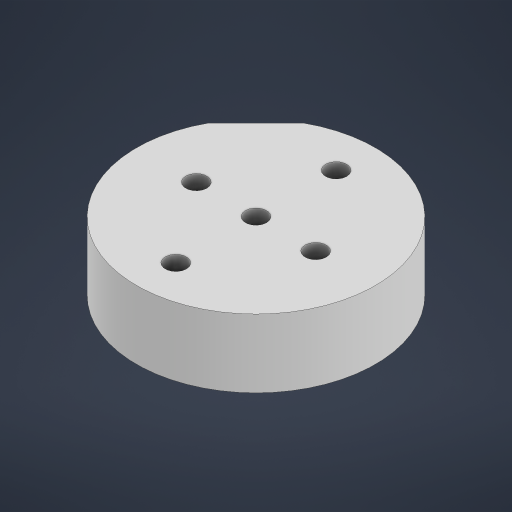
# Autodesk Inventor part: Pulley-35
Saved by Autodesk Inventor 2023 (Build 270158000, 158)
## iProperties
Created: 2023-09-04
Part Number: Pulley-35
Material: Generic
Document SubType Name: Modeling
Designer: Abhinav
Density: 1 g/cm^3
Appearance: Default
Author: Abhinav
Autodesk Inventor part; units mm, degrees
ref_plane "YZ Plane" through (0, 0, 0) normal (1, 0, 0) x (0, 1, 0)
ref_plane "XZ Plane" through (0, 0, 0) normal (0, 1, 0) x (-1, 0, 0)
ref_plane "XY Plane" through (0, 0, 0) normal (0, 0, 1) x (1, 0, 0)
sketch "Sketch1" plane through (0, 0, 0) normal (0, 1, 0) x (-1, 0, 0)
  line L0 (0, 0) -> (0, -11.75) construction
  circle A0 centre (0, -11.75) radius 1.55
  line L1 (0, 0) -> (8.75, 0) construction
  circle A1 centre (8.75, 0) radius 1.55
  circle A2 centre (0, 11.75) radius 1.55
  circle A3 centre (-8.75, 0) radius 1.55
  arc A4 (15.3686, -8.37) -> (8.37, -15.3686) centre (0, 0) ccw
  line L2 (0, 0) -> (12.3744, -12.3744) construction
  line L3 (0, 0) -> (17.5, 0) construction
  circle A5 centre (12.3744, -12.3744) radius 5 construction
  line L4 (15.3686, -8.37) -> (8.37, -15.3686)
  circle A6 centre (0, 0) radius 1.55
  dimension "d0" = 11.75
  dimension "d1" = 3.1
  dimension "d2" = 35
  dimension "d3" = 8.75
  dimension "d4" = 45
  dimension "d5" = 10
  constraints: 10 end point, 7 centre point, 5 coincident, 4 point on circle, 2 equal radius, 2 horizontal, 2 symmetric about line, 1 equal length, 1 vertical, 2 other
  measures "d0" distance of L0.start L0.end
  measures "d1" diameter of A0
  measures "d2" diameter of A4
  measures "d3" distance of L0.start L1.end
  measures "d4" angle of L2 L3
  measures "d5" diameter of A5
extrude "Extrusion1" add sketch "Sketch1" along normal blind 10
sketch "Sketch2" plane through (-15.3686, 0, -8.37) normal (-0.7071, 0, -0.7071) x (-0.7071, 0, 0.7071)
  line L0 (-9.8974, 10) -> (0, 10) construction
  line L1 (-9.8974, 0) -> (0, 0) construction
  line L2 (0, 10) -> (-9.8974, 0) construction
  circle A0 centre (-4.9487, 5) radius 1.5
  point P0 (-4.9487, 0)
  dimension "d9" = 3
  constraints: 2 end point, 1 centre point, 1 midpoint
  measures "d9" diameter of A0
extrude "Extrusion2" add sketch "Sketch2" along normal blind 5
body "Solid1"
